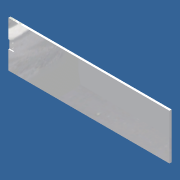
# Autodesk Inventor part: top panel for hinge left
Saved by Autodesk Inventor 2012 (Build 160160000, 160)
## iProperties
Created: 2012-02-06
Part Number: top panel for hinge left
Material: Default
Document SubType Name: Modeling
Designer: Allison Garza
Density: 1 g/cm^3
Author: Allison Garza
Autodesk Inventor part; units mm, degrees
ref_plane "YZ Plane" through (0, 0, 0) normal (1, 0, 0) x (0, 1, 0)
ref_plane "XZ Plane" through (0, 0, 0) normal (0, 1, 0) x (-1, 0, 0)
ref_plane "XY Plane" through (0, 0, 0) normal (0, 0, 1) x (1, 0, 0)
sketch "Sketch1" plane through (0, 0, 0) normal (0, 0, 1) x (1, 0, 0)
  line L0 (-35.8824, 13.1092) -> (434.0176, 13.1092)
  line L1 (434.0176, 13.1092) -> (434.0176, -120.2408)
  line L2 (434.0176, -120.2408) -> (-35.8824, -120.2408)
  line L3 (-35.8824, -120.2408) -> (-35.8824, 13.1092)
  point P0 (0, 0)
  dimension "d0" = 469.9
  dimension "d1" = 133.35
  constraints: 8 end point, 2 parallel, 1 horizontal, 1 perpendicular
  measures "d0" distance of L0.start L0.end
  measures "d1" distance of L2.end L0.start
extrude "Extrusion1" add sketch "Sketch1" along normal blind 6.35
sketch "Sketch2" plane through (0, 0, 6.35) normal (0, 0, 1) x (1, 0, 0)
  line L0 (434.0176, 13.1092) -> (434.0176, -120.2408) projected
  line L1 (434.0176, -40.8658) -> (418.1426, -40.8658)
  line L2 (418.1426, -40.8658) -> (418.1426, -66.2658)
  line L3 (418.1426, -66.2658) -> (434.0176, -66.2658)
  line L4 (434.0176, -66.2658) -> (434.0176, -40.8658)
  line L5 (-35.8824, 13.1092) -> (434.0176, 13.1092) projected
  line L6 (-35.8824, -120.2408) -> (-35.8824, 13.1092) projected
  line L7 (434.0176, -120.2408) -> (-35.8824, -120.2408) projected
  line L8 (199.0676, 13.1092) -> (199.0676, -120.2408)
  line L9 (-35.8824, -40.8658) -> (-20.0074, -40.8658)
  line L10 (-20.0074, -40.8658) -> (-20.0074, -66.2658)
  line L11 (-20.0074, -66.2658) -> (-35.8824, -66.2658)
  line L12 (-35.8824, -66.2658) -> (-35.8824, -40.8658)
  point P0 (0, 0)
  dimension "d4" = 15.875
  dimension "d5" = 25.4
  dimension "d6" = 53.975
  dimension "d16" = 234.95
  constraints: 18 end point, 4 symmetric about line, 3 parallel, 2 midpoint, 1 horizontal, 1 perpendicular, 1 point on line
  measures "d4" distance of L1.start L1.end
  measures "d5" distance of L1.end L2.end
  measures "d6" distance of L0.start L1.start
  measures "d16" distance of L6.start L8.end
ref_plane "Work Plane1" through (0, 0, 3.175) normal (0, 0, 1) x (1, 0, 0)
extrude "Extrusion4" cut sketch "Sketch2" against normal blind 3.175 contours L9 L10 L11 L6
sketch "Sketch4" plane through (0, 0, 3.175) normal (0, 0, 1) x (1, 0, 0)
  line L0 (-20.0074, -66.2658) -> (-20.0074, -40.8658) projected
  line L1 (-20.0074, -40.8658) -> (-35.8824, -40.8658) projected
  circle A0 centre (-26.3574, -47.2158) radius 1.5875
  circle A1 centre (-26.3574, -59.9158) radius 1.5875
  point P0 (0, 0)
  dimension "d19" = 6.35
  dimension "d20" = 12.7
  dimension "d21" = 6.35
  dimension "d22" = 3.175
  dimension "d23" = 3.175
  constraints: 2 centre point, 1 vertical alignment
  measures "d19" distance from line of L0 A0.centre
  measures "d20" distance of A0.centre A1.centre
  measures "d21" distance from line of L1 A0.centre
  measures "d22" diameter of A0
  measures "d23" diameter of A1
extrude "Extrusion5" cut sketch "Sketch4" against normal blind 3.175
body "Solid1"
